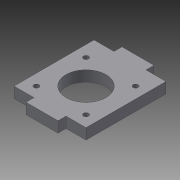
# Autodesk Inventor part: Frame_Lower_Plate_Motor
Saved by Autodesk Inventor 2014 (Build 180170000, 170)
## iProperties
Created: 2014-08-25
Part Number: Frame_Lower_Plate_Motor
Material: Generic
Document SubType Name: Modeling
Designer: ThatOtherGuy
Density: 1 g/cm^3
Appearance: Default
Author: ThatOtherGuy
Autodesk Inventor part; units mm, degrees
ref_plane "YZ Plane" through (0, 0, 0) normal (1, 0, 0) x (0, 1, 0)
ref_plane "XZ Plane" through (0, 0, 0) normal (0, 1, 0) x (-1, 0, 0)
ref_plane "XY Plane" through (0, 0, 0) normal (0, 0, 1) x (1, 0, 0)
sketch "Sketch1" plane through (0, 0, 0) normal (0, 0, 1) x (1, 0, 0)
  line L0 (0, 0) -> (12.5, 0)
  line L1 (12.5, 0) -> (12.5, -5)
  line L2 (12.5, -5) -> (32.5, -5)
  line L3 (32.5, -5) -> (32.5, 0)
  line L4 (32.5, 0) -> (45, 0)
  line L5 (45, 0) -> (45, 50)
  line L6 (45, 50) -> (32.5, 50)
  line L7 (32.5, 50) -> (32.5, 55)
  line L8 (32.5, 55) -> (12.5, 55)
  line L9 (12.5, 55) -> (12.5, 50)
  line L10 (12.5, 50) -> (0, 50)
  line L11 (0, 50) -> (0, 0)
  circle A0 centre (22.5, 22.5) radius 12.5
  circle A1 centre (7, 38) radius 1.6
  circle A2 centre (38, 38) radius 1.6
  circle A3 centre (38, 7) radius 1.6
  circle A4 centre (7, 7) radius 1.6
  point P0 (22.5, 55)
  dimension "d0" = 20
  dimension "d1" = 50
  dimension "d2" = 45
  dimension "d3" = 5
  dimension "d4" = 25
  dimension "d5" = 3.2
  dimension "d6" = 31
  dimension "d7" = 31
  dimension "d8" = 15.5
  dimension "d9" = 15.5
  dimension "d12" = 22.5
  constraints: 24 end point, 8 parallel, 6 equal length, 5 centre point, 3 equal radius, 3 vertical alignment, 2 collinear, 2 horizontal alignment, 1 horizontal, 1 midpoint, 1 perpendicular
  measures "d0" distance of L7.end L8.end
  measures "d1" distance of L10.end L0.start
  measures "d2" distance between parallel lines of L11 L5
  measures "d3" distance of L6.end L7.end
  measures "d4" diameter of A0
  measures "d5" diameter of A1
  measures "d6" distance of A4.centre A1.centre
  measures "d7" distance of A2.centre A1.centre
  measures "d8" horizontal distance of A0.centre A3.centre
  measures "d9" horizontal distance of A0.centre A3.centre
  measures "d12" distance from line of L0 A0.centre
extrude "Extrusion1" add sketch "Sketch1" along normal blind 6.731
equation "\"d7\" = d6"
equation "\"d8\" = 0.5 * d6"
equation "\"d9\" = 0.5 * d6"
equation "\"d10\" = THICKB"
equation "\"THICKA\" = 3.175"
equation "\"THICKB\" = 6.731"
equation "\"THICKC\" = 12.7"
equation "\"BALLDIA\" = 12"
equation "\"MAGDIA\" = 9.5"
equation "\"THICKPLY\" = 5"
body "Solid1"
